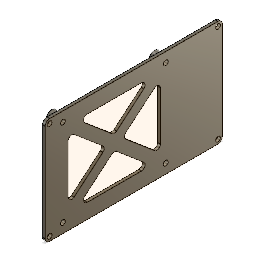
3dp-rock64-card v18 (Autodesk Fusion 360 design; units mm, degrees)
Autodesk Fusion 360 part; units mm, degrees
sketch "Sketch1" plane through (0, 0, 0) normal (1, 0, 0) x (0, 0, -1)
  line L0 (-50, 30) -> (50, 30)
  line L1 (50, 30) -> (50, -30)
  line L2 (50, -30) -> (-50, -30)
  line L3 (-50, -30) -> (-50, 30)
  line L4 (-50, 30) -> (50, -30) construction
  dimension "d1" = 100
  dimension "d2" = 60
extrude "Extrude1" add sketch "Sketch1" along normal blind 1.6002
sketch "Sketch2" plane through (1.6002, 0, 0) normal (1, 0, 0) x (0, 0, -1)
  line L0 (-50, -30) -> (50, -30)
  line L1 (50, -30) -> (50, 30)
  line L2 (50, 30) -> (-50, 30)
  line L3 (-50, 30) -> (-50, -30)
  line L4 (-50, 0) -> (50, 0) construction
  circle A0 centre (-40, 24.5) radius 1.375
  line L5 (-11, 30) -> (-11, -30) construction
  circle A1 centre (-40, -24.5) radius 1.375
  circle A2 centre (18, 24.5) radius 1.375
  circle A3 centre (18, -24.5) radius 1.375
  arc A4 (47.5, -30) -> (50, -27.5) centre (47.5, -27.5) ccw
  line L6 (50, -27.5) -> (50, 27.5)
  arc A5 (50, 27.5) -> (47.5, 30) centre (47.5, 27.5) ccw
  line L7 (47.5, 30) -> (-47.5, 30)
  arc A6 (-47.5, 30) -> (-50, 27.5) centre (-47.5, 27.5) ccw
  line L8 (-50, 27.5) -> (-50, -27.5)
  arc A7 (-50, -27.5) -> (-47.5, -30) centre (-47.5, -27.5) ccw
  line L9 (-47.5, -30) -> (47.5, -30)
  circle A8 centre (18, 24.5) radius 1.375
  circle A9 centre (18, -24.5) radius 1.375
  circle A10 centre (-40, 24.5) radius 1.375
  circle A11 centre (-40, -24.5) radius 1.375
  line L10 (-37, -13.7304) -> (-37, 13.7304)
  arc A12 (-33.7093, 15.2582) -> (-37, 13.7304) centre (-35, 13.7304) ccw
  line L11 (-33.7093, 15.2582) -> (-17.457, 1.5278)
  arc A13 (-17.457, -1.5278) -> (-17.457, 1.5278) centre (-18.7477, 0) ccw
  line L12 (-17.457, -1.5278) -> (-33.7093, -15.2582)
  arc A14 (-37, -13.7304) -> (-33.7093, -15.2582) centre (-35, -13.7304) ccw
  line L13 (-4.543, 1.5278) -> (11.7093, 15.2582)
  arc A15 (15, 13.7304) -> (11.7093, 15.2582) centre (13, 13.7304) ccw
  line L14 (15, 13.7304) -> (15, -13.7304)
  arc A16 (11.7093, -15.2582) -> (15, -13.7304) centre (13, -13.7304) ccw
  line L15 (11.7093, -15.2582) -> (-4.543, -1.5278)
  arc A17 (-4.543, 1.5278) -> (-4.543, -1.5278) centre (-3.2523, 0) ccw
  line L16 (-26.3339, 21.5) -> (4.3339, 21.5)
  arc A18 (5.6246, 17.9722) -> (4.3339, 21.5) centre (4.3339, 19.5) ccw
  line L17 (5.6246, 17.9722) -> (-9.7093, 5.0177)
  arc A19 (-12.2907, 5.0177) -> (-9.7093, 5.0177) centre (-11, 6.5455) ccw
  line L18 (-12.2907, 5.0177) -> (-27.6246, 17.9722)
  arc A20 (-26.3339, 21.5) -> (-27.6246, 17.9722) centre (-26.3339, 19.5) ccw
  line L19 (4.3339, -21.5) -> (-26.3339, -21.5)
  arc A21 (-27.6246, -17.9722) -> (-26.3339, -21.5) centre (-26.3339, -19.5) ccw
  line L20 (-27.6246, -17.9722) -> (-12.2907, -5.0177)
  arc A22 (-9.7093, -5.0177) -> (-12.2907, -5.0177) centre (-11, -6.5455) ccw
  line L21 (-9.7093, -5.0177) -> (5.6246, -17.9722)
  arc A23 (4.3339, -21.5) -> (5.6246, -17.9722) centre (4.3339, -19.5) ccw
  arc A24 (47.5, -30) -> (50, -27.5) centre (47.5, -27.5) ccw
  line L22 (50, -27.5) -> (50, 27.5)
  arc A25 (50, 27.5) -> (47.5, 30) centre (47.5, 27.5) ccw
  line L23 (47.5, 30) -> (-47.5, 30)
  arc A26 (-47.5, 30) -> (-50, 27.5) centre (-47.5, 27.5) ccw
  line L24 (-50, 27.5) -> (-50, -27.5)
  arc A27 (-50, -27.5) -> (-47.5, -30) centre (-47.5, -27.5) ccw
  line L25 (-47.5, -30) -> (47.5, -30)
  circle A28 centre (18, 24.5) radius 1.375
  circle A29 centre (18, -24.5) radius 1.375
  circle A30 centre (-40, 24.5) radius 1.375
  circle A31 centre (-40, -24.5) radius 1.375
  circle A32 centre (47.5, 27.5) radius 1.35
  circle A33 centre (47.5, -27.5) radius 1.35
  circle A34 centre (-47.5, 27.5) radius 1.35
  circle A35 centre (-47.5, -27.5) radius 1.35
  line L26 (-37, -13.7304) -> (-37, 13.7304)
  arc A36 (-33.7093, 15.2582) -> (-37, 13.7304) centre (-35, 13.7304) ccw
  line L27 (-33.7093, 15.2582) -> (-17.457, 1.5278)
  arc A37 (-17.457, -1.5278) -> (-17.457, 1.5278) centre (-18.7477, 0) ccw
  line L28 (-17.457, -1.5278) -> (-33.7093, -15.2582)
  arc A38 (-37, -13.7304) -> (-33.7093, -15.2582) centre (-35, -13.7304) ccw
  line L29 (-4.543, 1.5278) -> (11.7093, 15.2582)
  arc A39 (15, 13.7304) -> (11.7093, 15.2582) centre (13, 13.7304) ccw
  line L30 (15, 13.7304) -> (15, -13.7304)
  arc A40 (11.7093, -15.2582) -> (15, -13.7304) centre (13, -13.7304) ccw
  line L31 (11.7093, -15.2582) -> (-4.543, -1.5278)
  arc A41 (-4.543, 1.5278) -> (-4.543, -1.5278) centre (-3.2523, 0) ccw
  line L32 (-26.3339, 21.5) -> (4.3339, 21.5)
  arc A42 (5.6246, 17.9722) -> (4.3339, 21.5) centre (4.3339, 19.5) ccw
  line L33 (5.6246, 17.9722) -> (-9.7093, 5.0177)
  arc A43 (-12.2907, 5.0177) -> (-9.7093, 5.0177) centre (-11, 6.5455) ccw
  line L34 (-12.2907, 5.0177) -> (-27.6246, 17.9722)
  arc A44 (-26.3339, 21.5) -> (-27.6246, 17.9722) centre (-26.3339, 19.5) ccw
  line L35 (4.3339, -21.5) -> (-26.3339, -21.5)
  arc A45 (-27.6246, -17.9722) -> (-26.3339, -21.5) centre (-26.3339, -19.5) ccw
  line L36 (-27.6246, -17.9722) -> (-12.2907, -5.0177)
  arc A46 (-9.7093, -5.0177) -> (-12.2907, -5.0177) centre (-11, -6.5455) ccw
  line L37 (-9.7093, -5.0177) -> (5.6246, -17.9722)
  arc A47 (4.3339, -21.5) -> (5.6246, -17.9722) centre (4.3339, -19.5) ccw
  arc A48 (47.5, -30) -> (50, -27.5) centre (47.5, -27.5) ccw
  line L38 (50, -27.5) -> (50, 27.5)
  arc A49 (50, 27.5) -> (47.5, 30) centre (47.5, 27.5) ccw
  line L39 (47.5, 30) -> (-47.5, 30)
  arc A50 (-47.5, 30) -> (-50, 27.5) centre (-47.5, 27.5) ccw
  line L40 (-50, 27.5) -> (-50, -27.5)
  arc A51 (-50, -27.5) -> (-47.5, -30) centre (-47.5, -27.5) ccw
  line L41 (-47.5, -30) -> (47.5, -30)
  circle A52 centre (18, 24.5) radius 1.375
  circle A53 centre (18, -24.5) radius 1.375
  circle A54 centre (-40, 24.5) radius 1.375
  circle A55 centre (-40, -24.5) radius 1.375
  circle A56 centre (-47.5, 27.5) radius 1.35
  circle A57 centre (-47.5, -27.5) radius 1.35
  circle A58 centre (47.5, 27.5) radius 1.35
  circle A59 centre (47.5, -27.5) radius 1.35
  line L42 (37, 13.7304) -> (37, -13.7304)
  arc A60 (33.7093, -15.2582) -> (37, -13.7304) centre (35, -13.7304) ccw
  line L43 (33.7093, -15.2582) -> (17.457, -1.5278)
  arc A61 (17.457, 1.5278) -> (17.457, -1.5278) centre (18.7477, 0) ccw
  line L44 (17.457, 1.5278) -> (33.7093, 15.2582)
  arc A62 (37, 13.7304) -> (33.7093, 15.2582) centre (35, 13.7304) ccw
  line L45 (-11.7093, 15.2582) -> (4.543, 1.5278)
  arc A63 (4.543, -1.5278) -> (4.543, 1.5278) centre (3.2523, 0) ccw
  line L46 (4.543, -1.5278) -> (-11.7093, -15.2582)
  arc A64 (-15, -13.7304) -> (-11.7093, -15.2582) centre (-13, -13.7304) ccw
  line L47 (-15, -13.7304) -> (-15, 13.7304)
  arc A65 (-11.7093, 15.2582) -> (-15, 13.7304) centre (-13, 13.7304) ccw
  line L48 (-4.3339, 21.5) -> (26.3339, 21.5)
  arc A66 (27.6246, 17.9722) -> (26.3339, 21.5) centre (26.3339, 19.5) ccw
  line L49 (27.6246, 17.9722) -> (12.2907, 5.0177)
  arc A67 (9.7093, 5.0177) -> (12.2907, 5.0177) centre (11, 6.5455) ccw
  line L50 (9.7093, 5.0177) -> (-5.6246, 17.9722)
  arc A68 (-4.3339, 21.5) -> (-5.6246, 17.9722) centre (-4.3339, 19.5) ccw
  line L51 (26.3339, -21.5) -> (-4.3339, -21.5)
  arc A69 (-5.6246, -17.9722) -> (-4.3339, -21.5) centre (-4.3339, -19.5) ccw
  line L52 (-5.6246, -17.9722) -> (9.7093, -5.0177)
  arc A70 (12.2907, -5.0177) -> (9.7093, -5.0177) centre (11, -6.5455) ccw
  line L53 (12.2907, -5.0177) -> (27.6246, -17.9722)
  arc A71 (26.3339, -21.5) -> (27.6246, -17.9722) centre (26.3339, -19.5) ccw
  circle A72 centre (-18, 24.5) radius 1.375
  circle A73 centre (-18, -24.5) radius 1.375
  circle A74 centre (40, 24.5) radius 1.375
  circle A75 centre (40, -24.5) radius 1.375
  arc A76 (-50, -27.5) -> (-47.5, -30) centre (-47.5, -27.5) ccw
  line L54 (-47.5, -30) -> (47.5, -30)
  arc A77 (47.5, -30) -> (50, -27.5) centre (47.5, -27.5) ccw
  line L55 (50, -27.5) -> (50, 27.5)
  arc A78 (50, 27.5) -> (47.5, 30) centre (47.5, 27.5) ccw
  line L56 (47.5, 30) -> (-47.5, 30)
  arc A79 (-47.5, 30) -> (-50, 27.5) centre (-47.5, 27.5) ccw
  line L57 (-50, 27.5) -> (-50, -27.5)
  dimension "d5" = 58
  dimension "d6" = 49
  dimension "d7" = 2.75
  dimension "d8" = 10
  measures "d5" distance of origin
  measures "d7" diameter of A0
extrude "Extrude2" cut sketch "Sketch2" against normal through all contours A0 A10 A30 A54 | A1 A11 A31 A55 | A2 A8 A28 A52 | A3 A9 A29 A53
fillet "Fillet1" radius 2.5 4 edges at (0.8001, 30, -50) (0.8001, 30, 50) (0.8001, -30, 50) (0.8001, -30, -50)
sketch "Sketch4" plane through (1.6002, 0, 0) normal (1, 0, 0) x (0, 0, -1)
  arc A0 (47.5, -30) -> (50, -27.5) centre (47.5, -27.5) ccw
  line L0 (50, -27.5) -> (50, 27.5)
  arc A1 (50, 27.5) -> (47.5, 30) centre (47.5, 27.5) ccw
  line L1 (47.5, 30) -> (-47.5, 30)
  arc A2 (-47.5, 30) -> (-50, 27.5) centre (-47.5, 27.5) ccw
  line L2 (-50, 27.5) -> (-50, -27.5)
  arc A3 (-50, -27.5) -> (-47.5, -30) centre (-47.5, -27.5) ccw
  line L3 (-47.5, -30) -> (47.5, -30)
  circle A4 centre (18, 24.5) radius 1.375
  circle A5 centre (18, -24.5) radius 1.375
  circle A6 centre (-40, 24.5) radius 1.375
  circle A7 centre (-40, -24.5) radius 1.375
  line L4 (-40, 24.5) -> (18, 24.5)
  line L5 (18, 24.5) -> (-40, -24.5)
  line L6 (-40, -24.5) -> (18, -24.5)
  line L7 (18, -24.5) -> (-40, 24.5)
  line L8 (-40, 24.5) -> (-40, -24.5)
  line L9 (18, 24.5) -> (18, -24.5)
  line L10 (-11, 3.9273) -> (-31.8004, 21.5)
  line L11 (-31.8004, 21.5) -> (9.8004, 21.5)
  line L12 (9.8004, 21.5) -> (-11, 3.9273)
  line L13 (9.8004, -21.5) -> (-11, -3.9273)
  line L14 (-11, -3.9273) -> (-31.8004, -21.5)
  line L15 (-31.8004, -21.5) -> (9.8004, -21.5)
  dimension "d12" = 3
  dimension "d13" = 3
  measures "d12" distance of L7
  measures "d13" distance of L7
extrude "Extrude3" cut sketch "Sketch4" against normal through all contours L10 L11 L12 | L13 L14 L15
sketch "Sketch6" plane through (1.6002, 0, 0) normal (1, 0, 0) x (0, 0, -1)
  line L0 (-40, 24.5) -> (-40, -24.5)
  line L1 (18, -24.5) -> (-40, 24.5)
  line L2 (18, 24.5) -> (-40, -24.5)
  line L3 (18, 24.5) -> (18, -24.5)
  line L4 (-15.6486, 0) -> (-37, 18.0382)
  line L5 (-37, 18.0382) -> (-37, -18.0382)
  line L6 (-15.6486, 0) -> (-37, -18.0382)
  line L7 (15, 18.0382) -> (-6.3514, 0)
  line L8 (15, 18.0382) -> (15, -18.0382)
  line L9 (15, -18.0382) -> (-6.3514, 0)
  dimension "d15" = 3
  dimension "d16" = 3
  measures "d15" distance of L1
  measures "d16" distance of L2
extrude "Extrude4" cut sketch "Sketch6" against normal through all contours L4 L5 L6 | L7 L8 L9
fillet "Fillet2" radius 2 12 edges at (0.8001, 18.0382, 37) (0.8001, -3.9273, 11) (0.8001, 21.5, 31.8004) (0.8001, 21.5, -9.8004) (0.8001, 3.9273, 11) (0.8001, -18.0382, -15) (0.8001, 18.0382, -15) (0.8001, -21.5, -9.8004) (0.8001, 0, 15.6486) (0.8001, 0, 6.3514) (0.8001, -18.0382, 37) (0.8001, -21.5, 31.8004)
sketch "Sketch7" plane through (1.6002, 0, 0) normal (1, 0, 0) x (0, 0, -1)
  line L0 (-37, -13.7304) -> (-37, 13.7304)
  arc A0 (-33.7093, 15.2582) -> (-37, 13.7304) centre (-35, 13.7304) ccw
  line L1 (-33.7093, 15.2582) -> (-17.457, 1.5278)
  arc A1 (-17.457, -1.5278) -> (-17.457, 1.5278) centre (-18.7477, 0) ccw
  line L2 (-17.457, -1.5278) -> (-33.7093, -15.2582)
  arc A2 (-37, -13.7304) -> (-33.7093, -15.2582) centre (-35, -13.7304) ccw
  line L3 (-4.543, 1.5278) -> (11.7093, 15.2582)
  arc A3 (15, 13.7304) -> (11.7093, 15.2582) centre (13, 13.7304) ccw
  line L4 (15, 13.7304) -> (15, -13.7304)
  arc A4 (11.7093, -15.2582) -> (15, -13.7304) centre (13, -13.7304) ccw
  line L5 (11.7093, -15.2582) -> (-4.543, -1.5278)
  arc A5 (-4.543, 1.5278) -> (-4.543, -1.5278) centre (-3.2523, 0) ccw
  line L6 (-26.3339, 21.5) -> (4.3339, 21.5)
  arc A6 (5.6246, 17.9722) -> (4.3339, 21.5) centre (4.3339, 19.5) ccw
  line L7 (5.6246, 17.9722) -> (-9.7093, 5.0177)
  arc A7 (-12.2907, 5.0177) -> (-9.7093, 5.0177) centre (-11, 6.5455) ccw
  line L8 (-12.2907, 5.0177) -> (-27.6246, 17.9722)
  arc A8 (-26.3339, 21.5) -> (-27.6246, 17.9722) centre (-26.3339, 19.5) ccw
  line L9 (4.3339, -21.5) -> (-26.3339, -21.5)
  arc A9 (-27.6246, -17.9722) -> (-26.3339, -21.5) centre (-26.3339, -19.5) ccw
  line L10 (-27.6246, -17.9722) -> (-12.2907, -5.0177)
  arc A10 (-9.7093, -5.0177) -> (-12.2907, -5.0177) centre (-11, -6.5455) ccw
  line L11 (-9.7093, -5.0177) -> (5.6246, -17.9722)
  arc A11 (4.3339, -21.5) -> (5.6246, -17.9722) centre (4.3339, -19.5) ccw
  arc A12 (47.5, -30) -> (50, -27.5) centre (47.5, -27.5) ccw
  line L12 (50, -27.5) -> (50, 27.5)
  arc A13 (50, 27.5) -> (47.5, 30) centre (47.5, 27.5) ccw
  line L13 (47.5, 30) -> (-47.5, 30)
  arc A14 (-47.5, 30) -> (-50, 27.5) centre (-47.5, 27.5) ccw
  line L14 (-50, 27.5) -> (-50, -27.5)
  arc A15 (-50, -27.5) -> (-47.5, -30) centre (-47.5, -27.5) ccw
  line L15 (-47.5, -30) -> (47.5, -30)
  circle A16 centre (18, 24.5) radius 1.375
  circle A17 centre (18, -24.5) radius 1.375
  circle A18 centre (-40, 24.5) radius 1.375
  circle A19 centre (-40, -24.5) radius 1.375
  circle A20 centre (47.5, 27.5) radius 1.35
  circle A21 centre (47.5, -27.5) radius 1.35
  circle A22 centre (-47.5, -27.5) radius 1.35
  circle A23 centre (-47.5, 27.5) radius 1.35
  line L16 (0, 30) -> (0, -30) construction
  circle A24 centre (0, 27.5) radius 1.35
  line L17 (-50, 0) -> (50, 0) construction
  circle A25 centre (0, -27.5) radius 1.35
  dimension "d19" = 2.7
  dimension "d24" = 2.5
  measures "d19" diameter of A23
extrude "Extrude5" cut sketch "Sketch7" against normal through all contours A20 | A21 | A22 | A23
sketch "Sketch8" plane through (1.6002, 0, 0) normal (1, 0, 0) x (0, 0, -1)
  circle A0 centre (47.5, 27.5) radius 1.35
  circle A1 centre (47.5, -27.5) radius 1.35
  circle A2 centre (-47.5, 27.5) radius 1.35
  circle A3 centre (-47.5, -27.5) radius 1.35
  line L0 (-37, -13.7304) -> (-37, 13.7304)
  arc A4 (-33.7093, 15.2582) -> (-37, 13.7304) centre (-35, 13.7304) ccw
  line L1 (-33.7093, 15.2582) -> (-17.457, 1.5278)
  arc A5 (-17.457, -1.5278) -> (-17.457, 1.5278) centre (-18.7477, 0) ccw
  line L2 (-17.457, -1.5278) -> (-33.7093, -15.2582)
  arc A6 (-37, -13.7304) -> (-33.7093, -15.2582) centre (-35, -13.7304) ccw
  line L3 (-4.543, 1.5278) -> (11.7093, 15.2582)
  arc A7 (15, 13.7304) -> (11.7093, 15.2582) centre (13, 13.7304) ccw
  line L4 (15, 13.7304) -> (15, -13.7304)
  arc A8 (11.7093, -15.2582) -> (15, -13.7304) centre (13, -13.7304) ccw
  line L5 (11.7093, -15.2582) -> (-4.543, -1.5278)
  arc A9 (-4.543, 1.5278) -> (-4.543, -1.5278) centre (-3.2523, 0) ccw
  line L6 (-26.3339, 21.5) -> (4.3339, 21.5)
  arc A10 (5.6246, 17.9722) -> (4.3339, 21.5) centre (4.3339, 19.5) ccw
  line L7 (5.6246, 17.9722) -> (-9.7093, 5.0177)
  arc A11 (-12.2907, 5.0177) -> (-9.7093, 5.0177) centre (-11, 6.5455) ccw
  line L8 (-12.2907, 5.0177) -> (-27.6246, 17.9722)
  arc A12 (-26.3339, 21.5) -> (-27.6246, 17.9722) centre (-26.3339, 19.5) ccw
  line L9 (4.3339, -21.5) -> (-26.3339, -21.5)
  arc A13 (-27.6246, -17.9722) -> (-26.3339, -21.5) centre (-26.3339, -19.5) ccw
  line L10 (-27.6246, -17.9722) -> (-12.2907, -5.0177)
  arc A14 (-9.7093, -5.0177) -> (-12.2907, -5.0177) centre (-11, -6.5455) ccw
  line L11 (-9.7093, -5.0177) -> (5.6246, -17.9722)
  arc A15 (4.3339, -21.5) -> (5.6246, -17.9722) centre (4.3339, -19.5) ccw
  arc A16 (47.5, -30) -> (50, -27.5) centre (47.5, -27.5) ccw
  line L12 (50, -27.5) -> (50, 27.5)
  arc A17 (50, 27.5) -> (47.5, 30) centre (47.5, 27.5) ccw
  line L13 (47.5, 30) -> (-47.5, 30)
  arc A18 (-47.5, 30) -> (-50, 27.5) centre (-47.5, 27.5) ccw
  line L14 (-50, 27.5) -> (-50, -27.5)
  arc A19 (-50, -27.5) -> (-47.5, -30) centre (-47.5, -27.5) ccw
  line L15 (-47.5, -30) -> (47.5, -30)
  circle A20 centre (18, 24.5) radius 1.375
  circle A21 centre (18, -24.5) radius 1.375
  circle A22 centre (-40, 24.5) radius 1.375
  circle A23 centre (-40, -24.5) radius 1.375
sketch "Sketch9" plane through (0, 0, 0) normal (-1, 0, 0) x (0, 0, 1)
  circle A0 centre (-47.5, 27.5) radius 1.35
  circle A1 centre (-47.5, -27.5) radius 1.35
  circle A2 centre (47.5, 27.5) radius 1.35
  circle A3 centre (47.5, -27.5) radius 1.35
  line L0 (37, 13.7304) -> (37, -13.7304)
  arc A4 (33.7093, -15.2582) -> (37, -13.7304) centre (35, -13.7304) ccw
  line L1 (33.7093, -15.2582) -> (17.457, -1.5278)
  arc A5 (17.457, 1.5278) -> (17.457, -1.5278) centre (18.7477, 0) ccw
  line L2 (17.457, 1.5278) -> (33.7093, 15.2582)
  arc A6 (37, 13.7304) -> (33.7093, 15.2582) centre (35, 13.7304) ccw
  line L3 (-11.7093, 15.2582) -> (4.543, 1.5278)
  arc A7 (4.543, -1.5278) -> (4.543, 1.5278) centre (3.2523, 0) ccw
  line L4 (4.543, -1.5278) -> (-11.7093, -15.2582)
  arc A8 (-15, -13.7304) -> (-11.7093, -15.2582) centre (-13, -13.7304) ccw
  line L5 (-15, -13.7304) -> (-15, 13.7304)
  arc A9 (-11.7093, 15.2582) -> (-15, 13.7304) centre (-13, 13.7304) ccw
  line L6 (-4.3339, 21.5) -> (26.3339, 21.5)
  arc A10 (27.6246, 17.9722) -> (26.3339, 21.5) centre (26.3339, 19.5) ccw
  line L7 (27.6246, 17.9722) -> (12.2907, 5.0177)
  arc A11 (9.7093, 5.0177) -> (12.2907, 5.0177) centre (11, 6.5455) ccw
  line L8 (9.7093, 5.0177) -> (-5.6246, 17.9722)
  arc A12 (-4.3339, 21.5) -> (-5.6246, 17.9722) centre (-4.3339, 19.5) ccw
  line L9 (26.3339, -21.5) -> (-4.3339, -21.5)
  arc A13 (-5.6246, -17.9722) -> (-4.3339, -21.5) centre (-4.3339, -19.5) ccw
  line L10 (-5.6246, -17.9722) -> (9.7093, -5.0177)
  arc A14 (12.2907, -5.0177) -> (9.7093, -5.0177) centre (11, -6.5455) ccw
  line L11 (12.2907, -5.0177) -> (27.6246, -17.9722)
  arc A15 (26.3339, -21.5) -> (27.6246, -17.9722) centre (26.3339, -19.5) ccw
  circle A16 centre (-18, 24.5) radius 1.375
  circle A17 centre (-18, -24.5) radius 1.375
  circle A18 centre (40, 24.5) radius 1.375
  circle A19 centre (40, -24.5) radius 1.375
  arc A20 (-50, -27.5) -> (-47.5, -30) centre (-47.5, -27.5) ccw
  line L12 (-47.5, -30) -> (47.5, -30)
  arc A21 (47.5, -30) -> (50, -27.5) centre (47.5, -27.5) ccw
  line L13 (50, -27.5) -> (50, 27.5)
  arc A22 (50, 27.5) -> (47.5, 30) centre (47.5, 27.5) ccw
  line L14 (47.5, 30) -> (-47.5, 30)
  arc A23 (-47.5, 30) -> (-50, 27.5) centre (-47.5, 27.5) ccw
  line L15 (-50, 27.5) -> (-50, -27.5)
  circle A24 centre (-18, 24.5) radius 3
  circle A25 centre (40, 24.5) radius 3
  circle A26 centre (40, -24.5) radius 3
  circle A27 centre (-18, -24.5) radius 3
  dimension "d25" = 6
  measures "d25" diameter of A24
extrude "Extrude6" add sketch "Sketch9" along normal blind 5 contours A24 | A25 | A26 | A27
fillet "Fillet3" radius 2 4 edges at (0, 25.5848, 37.203) (0, 25.5848, -20.797) (0, -23.4152, 37.203) (0, -23.4152, -20.797)
fillet "Fillet4" radius 0.25 8 edges at (-5, 24.9972, 38.718) (-5, 24.9972, -19.282) (-5, -24.0028, 38.718) (-5, -24.0028, -19.282) (-5, -25.5848, -20.797) (-5, 23.4152, -20.797) (-5, 23.4152, 37.203) (-5, -25.5848, 37.203)
